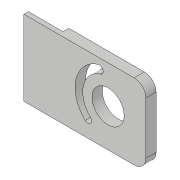
# Autodesk Inventor part: Lidar Sensor Case v4 Piece 3
Saved by Autodesk Inventor 2018.3 (Build 223284000, 284)
## iProperties
Created: 2019-03-27
Part Number: Lidar Sensor Case v4 Piece 3
Material: Generic
Document SubType Name: Modeling
Designer: aye06091
Mass: 12.4743 g
Surface Area: 69.2649 cm^2
Volume: 12.4743 cm^3
Density: 1 g/cm^3
Appearance: Default
Author: aye06091
Autodesk Inventor part; units mm, degrees
ref_plane "YZ Plane" through (0, 0, 0) normal (1, 0, 0) x (0, 1, 0)
ref_plane "XZ Plane" through (0, 0, 0) normal (0, 1, 0) x (-1, 0, 0)
ref_plane "XY Plane" through (0, 0, 0) normal (0, 0, 1) x (1, 0, 0)
sketch "Sketch1" plane through (0, 0, 0) normal (0, 0, 1) x (1, 0, 0)
  line L0 (0, 0) -> (66.675, 0)
  line L1 (66.675, 0) -> (66.675, -41.275)
  line L2 (66.675, -41.275) -> (0, -41.275)
  line L3 (0, -41.275) -> (0, 0)
  arc A0 (40.6531, -3.4261) -> (33.474, -33.5752) centre (46.0375, -20.6375) ccw
  arc A1 (41.8969, -7.4017) -> (36.376, -30.5868) centre (46.0375, -20.6375) ccw
  circle A2 centre (46.0375, -20.6375) radius 8.7948
  arc A3 (41.8969, -7.4017) -> (40.6531, -3.4261) centre (41.275, -5.4139) ccw
  arc A4 (33.474, -33.5752) -> (36.376, -30.5868) centre (34.925, -32.081) ccw
  dimension "d0" = 41.275
  dimension "d1" = 66.675
  dimension "d4" = 17.5895
  dimension "d5" = 20.6375
  dimension "d22" = 20.6375
  dimension "d23" = 25.4
  dimension "d24" = 31.75
  dimension "d54" = 2.0828
  dimension "d55" = 15.9512
  constraints: 10 point on circle, 8 end point, 5 centre point, 4 tangent, 3 coincident, 2 parallel, 1 horizontal, 1 perpendicular
  measures "d0" distance of L2.end L0.start
  measures "d1" distance of L0.start L0.end
  measures "d4" diameter of A2
  measures "d5" distance from line of L0 A0.centre
  measures "d22" distance from line of L1 A0.centre
  measures "d23" distance from line of L1 A3.centre
  measures "d24" distance from line of L1 A4.centre
  measures "d54" radius of A3
  measures "d55" distance of A1.centre A3.centre
extrude "Extrusion1" add sketch "Sketch1" against normal blind 5.6134
sketch "Sketch5" plane through (0, 0, -5.6134) normal (0, 0, -1) x (-1, 0, 0)
  line L0 (0, 0) -> (-66.675, 0) projected
  line L1 (-66.675, -41.275) -> (0, -41.275) projected
  line L2 (0, -41.275) -> (0, 0) projected
  line L3 (-18.8976, 0) -> (-15.875, 0)
  line L4 (-15.875, 0) -> (-15.875, -41.275)
  line L5 (-15.875, -41.275) -> (-18.8976, -41.275)
  line L6 (-18.8976, -41.275) -> (-18.8976, 0)
  line L7 (-18.8976, 0) -> (0, 0)
  line L8 (0, 0) -> (0, -3.175)
  line L9 (0, -3.175) -> (-18.8976, -3.175)
  line L10 (-18.8976, -3.175) -> (-18.8976, 0)
  line L11 (-15.875, -39.6875) -> (0, -39.6875)
  line L12 (0, -39.6875) -> (0, -37.5285)
  line L13 (0, -37.5285) -> (-15.875, -37.5285)
  line L14 (-15.875, -37.5285) -> (-15.875, -39.6875)
  dimension "d37" = 3.0226
  dimension "d38" = 15.875
  dimension "d39" = 3.175
  dimension "d43" = 1.5875
  dimension "d44" = 2.159
  constraints: 24 end point, 6 parallel, 5 point on line, 3 horizontal, 3 perpendicular
  measures "d37" distance between parallel lines of L4 L6
  measures "d38" distance between parallel lines of L2 L4
  measures "d39" distance between parallel lines of L0 L9
  measures "d43" distance between parallel lines of L1 L11
  measures "d44" distance between parallel lines of L13 L11
extrude "Extrusion5" cut sketch "Sketch5" against normal blind 3.175 contours L2 L9 L4 L0 | L4 L9 L6 L0 | L4 L1 L6 L9 | L2 L11 L4 L13
fillet "Fillet1" radius 6.35 2 edges at (66.675, 0, -2.8067) (66.675, -41.275, -2.8067)
body "Solid1"
